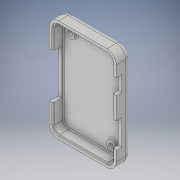
# Autodesk Inventor part: Bottom
Saved by Autodesk Inventor 2018.3 (Build 223284000, 284)
## iProperties
Created: 2018-10-08
Part Number: Bottom
Material: Generic
Document SubType Name: Modeling
Designer: birtj
Density: 1 g/cm^3
Appearance: Default
Author: birtj
Autodesk Inventor part; units mm, degrees
ref_plane "YZ Plane" through (0, 0, 0) normal (1, 0, 0) x (0, 1, 0)
ref_plane "XZ Plane" through (0, 0, 0) normal (0, 1, 0) x (-1, 0, 0)
ref_plane "XY Plane" through (0, 0, 0) normal (0, 0, 1) x (1, 0, 0)
sketch "OBJECT" plane through (0, 0, 0) normal (0, 0, 1) x (1, 0, 0)
  line L0 (177.8812, 243.8295) -> (177.8812, 295.7471)
  arc A0 (183.6724, 301.5383) -> (177.8812, 295.7471) centre (183.6724, 295.7471) ccw
  line L1 (183.6724, 301.5383) -> (213.492, 301.5383)
  arc A1 (219.2832, 295.7471) -> (213.492, 301.5383) centre (213.492, 295.7471) ccw
  line L2 (219.2832, 295.7471) -> (219.2832, 243.8295)
  arc A2 (213.492, 238.0383) -> (219.2832, 243.8295) centre (213.492, 243.8295) ccw
  line L3 (213.492, 238.0383) -> (183.6724, 238.0383)
  arc A3 (177.8812, 243.8295) -> (183.6724, 238.0383) centre (183.6724, 243.8295) ccw
  dimension "d2" = 63.5
  dimension "d3" = 41.402
  constraints: 8 end point, 8 point on circle, 4 centre point
  measures "d2" distance between parallel lines of L3 L1
  measures "d3" distance between parallel lines of L2 L0
extrude "Extrusion1" add sketch "OBJECT" along normal blind 8.9154
shell "Shell1" thickness 2.3622 removed faces 1 at (191.6819, 261.1354, 8.9154)
sketch "Sketch4" plane through (183.6724, 240.4005, 2.3622) normal (0, 0, 1) x (1, 0, 0)
  line L0 (29.8196, 61.1378) -> (0, 61.1378) construction
  line L1 (14.9098, 61.1378) -> (14.9098, -2.3622) construction
  line L2 (0, -2.3622) -> (29.8196, -2.3622) construction
  line L3 (-5.7912, 55.3466) -> (-5.7912, 3.429) construction
  line L4 (-5.7912, 29.3878) -> (35.6108, 29.3878) construction
  line L5 (35.6108, 3.429) -> (35.6108, 55.3466) construction
  circle A0 centre (27.6098, 5.6388) radius 2.921
  circle A1 centre (2.2098, 53.1368) radius 2.921
  dimension "d9" = 12.7
  dimension "d10" = 12.7
  dimension "d11" = 5.842
  dimension "d12" = 5.842
  dimension "d38" = 23.749
  dimension "d40" = 23.749
  constraints: 4 end point, 4 midpoint, 2 centre point, 2 coincident
  measures "d9" distance from line of L1 point (2.21, 53.137)
  measures "d10" distance from line of L1 point (27.61, 5.639)
  measures "d11" diameter of A0
  measures "d12" diameter of A1
  measures "d38" distance from line of L4 point (2.21, 53.137)
  measures "d40" distance from line of L4 point (27.61, 5.639)
extrude "Extrusion2" add sketch "Sketch4" along normal blind 1.778
sketch "Sketch5" plane through (185.8822, 293.5373, 4.1402) normal (0, 0, 1) x (1, 0, 0)
  circle A0 centre (25.4, -47.498) radius 2.921 projected
  point P0 (-185.8822, -293.5373)
  point P1 (0, 0)
  constraints: 1 coincident
hole "Hole1" at (185.8822, 293.5373, 4.1402) at (211.2822, 246.0393, 4.1402) direction (0, 0, -1) diameter 3.2766 end through all clearance for "Flat Head Machine Screw (82)" size "#4" standard "Ansi Unified Screw Threads"
fillet "Fillet1" radius 3.175 8 edges at (179.5774, 299.8421, 0) (177.8812, 269.7883, 0) (179.5774, 239.7345, 0) (198.5822, 238.0383, 0) (217.587, 239.7345, 0) (219.2832, 269.7883, 0) (217.587, 299.8421, 0) (198.5822, 301.5383, 0)
sketch "Sketch6" plane through (219.2832, 243.8295, 8.9154) normal (1, 0, 0) x (0, 0, -1)
  line L0 (0, 51.9176) -> (0, 0) projected
  line L1 (0, 45.0088) -> (3.429, 45.0088)
  line L2 (3.429, 45.0088) -> (3.429, 35.4838)
  line L3 (3.429, 35.4838) -> (0, 35.4838)
  line L4 (0, 35.4838) -> (0, 45.0088)
  line L5 (5.7404, 57.7088) -> (0, 57.7088) projected
  line L6 (0, 6.1468) -> (3.429, 6.1468)
  line L7 (3.429, 6.1468) -> (3.429, 22.0218)
  line L8 (3.429, 22.0218) -> (0, 22.0218)
  line L9 (0, 22.0218) -> (0, 6.1468)
  line L10 (5.7404, -5.7912) -> (0, -5.7912) projected
  point P0 (8.9154, -243.8295)
  dimension "d23" = 9.525
  dimension "d24" = 12.7
  dimension "d25" = 3.429
  dimension "d26" = 11.938
  dimension "d27" = 15.875
  dimension "d28" = 3.429
  constraints: 16 end point, 4 parallel, 2 horizontal, 2 perpendicular, 2 point on line
  measures "d23" distance of L1.end L2.end
  measures "d24" distance between parallel lines of L1 L5
  measures "d25" distance of L2.end L3.end
  measures "d26" distance between parallel lines of L6 L10
  measures "d27" distance of L6.end L7.end
  measures "d28" distance of L6.start L6.end
extrude "Extrusion3" cut sketch "Sketch6" against normal blind 2.54
sketch "Sketch7" plane through (177.8812, 243.8295, 8.9154) normal (-1, 0, 0) x (0, 0, 1)
  line L0 (0, 35.4838) -> (0, 22.0218) construction
  line L1 (-8.9154, 51.9176) -> (-8.9154, 0) construction
  line L2 (0, 39.9288) -> (-5.461, 39.9288)
  line L3 (-5.461, 39.9288) -> (-5.461, 11.9888)
  line L4 (-5.461, 11.9888) -> (0, 11.9888)
  line L5 (0, 11.9888) -> (0, 39.9288)
  line L6 (-5.7404, -5.7912) -> (0, -5.7912) projected
  line L7 (-5.7404, 57.7088) -> (0, 57.7088) projected
  point P0 (-8.9154, -243.8295)
  dimension "d31" = 5.461
  dimension "d32" = 27.94
  dimension "d35" = 63.5
  dimension "d36" = 17.78
  constraints: 8 end point, 2 parallel, 1 horizontal, 1 perpendicular
  measures "d31" distance of L4.end L3.end
  measures "d32" distance of L3.end L2.end
  measures "d35" distance between parallel lines of L6 L7
  measures "d36" distance between parallel lines of L7 L2
extrude "Extrusion4" cut sketch "Sketch7" against normal blind 2.54
sketch "Sketch8" plane through (0, 0, 0) normal (0, 0, -1) x (-1, 0, 0)
  circle A0 centre (-211.2822, 246.0393) radius 1.6383 projected
  circle A1 centre (-185.8822, 293.5373) radius 1.6383 projected
  constraints: 2 coincident
hole "Hole2" at (211.2822, 246.0393, 0) at (185.8822, 293.5373, 0) direction (0, 0, 1) diameter 3.2766 end through all countersink diameter 5.715 countersink angle 82 clearance for "Flat Head Machine Screw (82)" size "#4" standard "Ansi Unified Screw Threads"
lip "Lip1" kind groove height 0.762 width 0.762 edges at (180.2434, 289.7527, 8.9154) (181.2478, 298.1718, 8.9154) (198.5822, 299.1761, 8.9154) (215.9167, 298.1718, 8.9154) (216.921, 292.2927, 8.9154) guide face at (203.5522, 299.9635, 8.9154)
lip "Lip3" kind groove height 0.762 width 0.762 edges at (198.5822, 240.4005, 8.9154) (181.2478, 241.4048, 8.9154) (180.2434, 249.8239, 8.9154) (215.9167, 241.4048, 8.9154) (216.921, 246.9029, 8.9154) guide face at (203.5522, 238.8257, 8.9154)
lip "Lip4" kind groove height 0.762 width 0.762 edges at (216.921, 272.5823, 8.9154) guide face at (217.7084, 274.826, 8.9154)
fillet "Fillet2" radius 0.635 10 edges at (182.9612, 293.5373, 2.3622) (208.3612, 246.0393, 2.3622) (215.9167, 241.4048, 2.3622) (216.921, 269.7883, 2.3622) (215.9167, 298.1718, 2.3622) (198.5822, 299.1761, 2.3622) (181.2478, 298.1718, 2.3622) (180.2434, 269.7883, 2.3622) (181.2478, 241.4048, 2.3622) (198.5822, 240.4005, 2.3622)
equation "\"d36\" = -0.5 * d32 + 0.5 * d35"
body "Solid1"
